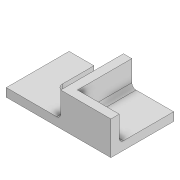
# Autodesk Inventor part: Laptop-ecke-l
Saved by Autodesk Inventor 2022 (Build 260153000, 153)
## iProperties
Created: 2024-04-12
Part Number: Laptop-ecke-l
Material: Generic
Document SubType Name: Modeling
Designer: LaptopJR
Density: 1 g/cm^3
Appearance: Default
Author: LaptopJR
## iProperties of the stored document Laptop-ecke-l_3DPrint.ipt
Created: 2024-04-12
Part Number: Laptop-ecke-l_3DPrint
Material: Generic
Document SubType Name: Modeling
Designer: LaptopJR
Density: 1 g/cm^3
Appearance: Default
Author: LaptopJR
Autodesk Inventor part; units mm, degrees
ref_plane "YZ Plane" through (0, 0, 0) normal (1, 0, 0) x (0, 1, 0)
ref_plane "XZ Plane" through (0, 0, 0) normal (0, 1, 0) x (-1, 0, 0)
ref_plane "XY Plane" through (0, 0, 0) normal (0, 0, 1) x (1, 0, 0)
sketch "Sketch1" plane through (0, 0, 0) normal (0, 1, 0) x (-1, 0, 0)
  line L0 (0, 0) -> (-50, 0)
  line L1 (-50, 0) -> (-50, -30)
  line L2 (0, -30) -> (0, 0)
  line L3 (-50, -15) -> (-15, -15) construction
  arc A0 (-11.9, -15) -> (-18.1, -15) centre (-15, -15) ccw
  line L4 (-11.9, -15) -> (-11.9, -30)
  line L5 (-18.1, -15) -> (-18.1, -30)
  line L6 (-50, -30) -> (-18.1, -30)
  line L7 (-11.9, -30) -> (0, -30)
  dimension "d0" = 35
  dimension "d1" = 6.2
  dimension "d2" = 30
  dimension "d3" = 50
  constraints: 16 end point, 5 perpendicular, 3 parallel, 2 horizontal, 2 point on circle, 1 centre point, 1 coincident, 1 midpoint, 1 point on line, 1 tangent
  measures "d0" distance of L3.start L3.end
  measures "d1" diameter of A0
  measures "d2" distance of L0.end L1.end
  measures "d3" distance of L0.start L0.end
extrude "Extrusion1" add sketch "Sketch1" along normal blind 4
sketch "Sketch3" plane through (0, 4, 0) normal (0, 1, 0) x (1, 0, 0)
  line L0 (50, 30) -> (18.1, 30) projected
  line L1 (30, 30) -> (30, 4)
  line L2 (30, 4) -> (50, 4)
  line L3 (0, 30) -> (0, 0) projected
  line L4 (26, 30) -> (26, 0)
  line L5 (0, 0) -> (50, 0) projected
  line L6 (50, 0) -> (50, 30) projected
  dimension "d12" = 30
  dimension "d13" = 4
  dimension "d14" = 4
  constraints: 6 end point, 3 point on line, 2 vertical, 1 perpendicular
  measures "d12" distance between parallel lines of L1 L3
  measures "d13" distance between parallel lines of L1 L4
  measures "d14" distance between parallel lines of L5 L2
extrude "Extrusion3" add sketch "Sketch3" along normal blind 12 contours L1 L2 L6 L5 L4 L0
fillet "Fillet2" radius 2 3 edges at (26, 4, -15) (30, 4, -17) (40, 4, -4)
body "Solid1"
